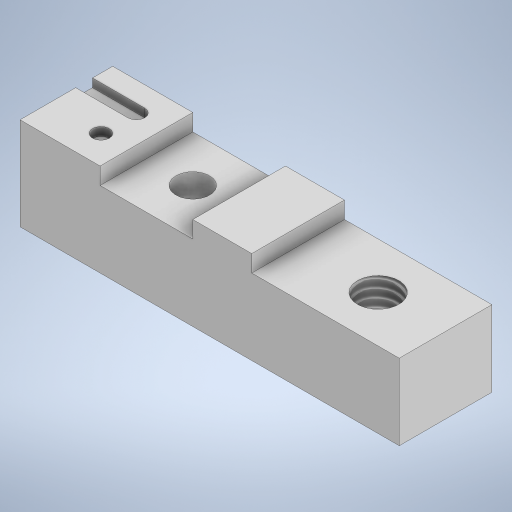
# Autodesk Inventor part: Hudson 1-55
Saved by Autodesk Inventor 2024.2 (Build 282272000, 272)
## iProperties
Created: 2024-10-06
Part Number: Hudson 1-55
Material: Genérico
Document SubType Name: Modeling
Designer: Monica Mora
Density: 1 g/cm^3
Appearance: Valor por defecto
Author: Monica Mora
Autodesk Inventor part; units mm, degrees
ref_plane "YZ Plane" through (0, 0, 0) normal (1, 0, 0) x (0, 1, 0)
ref_plane "XZ Plane" through (0, 0, 0) normal (0, 1, 0) x (-1, 0, 0)
ref_plane "XY Plane" through (0, 0, 0) normal (0, 0, 1) x (1, 0, 0)
sketch "Boceto1" plane through (0, 0, 0) normal (0, 0, 1) x (1, 0, 0)
  line L0 (0, 0) -> (-45, 0)
  line L1 (-45, 0) -> (-45, 11)
  line L2 (0, 9) -> (0, 0)
  line L3 (-35.5, 11) -> (-35.5, 9)
  line L4 (-35.5, 9) -> (-24.5, 9)
  line L5 (-24.5, 9) -> (-24.5, 11)
  line L6 (-17.5, 11) -> (-17.5, 9)
  line L7 (-17.5, 9) -> (0, 9)
  line L8 (-45, 11) -> (-35.5, 11)
  line L9 (-24.5, 11) -> (-17.5, 11)
  dimension "d0" = 9
  dimension "d1" = 11
  dimension "d2" = 9.5
  dimension "d3" = 7
  dimension "d4" = 17.5
  dimension "d5" = 11
  dimension "d6" = 2
  dimension "d7" = 2
  constraints: 20 end point, 5 perpendicular, 4 parallel, 2 point on line, 1 horizontal
  measures "d0" distance between parallel lines of L0 L7
  measures "d1" distance of L0.end L1.end
  measures "d2" distance of L1.end L3.start
  measures "d3" distance of L5.end L6.start
  measures "d4" distance of L6.end L2.start
  measures "d5" distance of L3.end L4.end
  measures "d6" distance of L3.start L3.end
  measures "d7" distance of L4.end L5.end
extrude "Extrusión1" add sketch "Boceto1" along normal blind 11
sketch "Boceto2" plane through (-45, 0, 0) normal (0, -1, 0) x (1, 0, 0)
  line L0 (0, 0) -> (45, 0) projected
  line L1 (45, 0) -> (45, 11) projected
  line L2 (0, 11) -> (45, 11) projected
  line L3 (0, 0) -> (0, 11) projected
  line L4 (45, 5.5) -> (0, 5.5) construction
  line L5 (45, 11) -> (27.5, 11) projected
  line L6 (37, 11) -> (37, 0) construction
  line L7 (15, 11) -> (15, 0) construction
  line L8 (0, 0) -> (45, 0) projected
  circle A0 centre (37, 5.5) radius 2.85
  circle A1 centre (15, 5.5) radius 4.5
  circle A2 centre (15, 5.5) radius 2
  dimension "d10" = 8
  dimension "d11" = 22
  dimension "d12" = 9
  dimension "d13" = 4
  dimension "d14" = 5.7
  constraints: 6 end point, 4 midpoint, 4 point on line, 3 centre point, 2 perpendicular, 1 coincident
  measures "d10" distance between parallel lines of L6 L1
  measures "d11" distance between parallel lines of L7 L6
  measures "d12" diameter of A1
  measures "d13" diameter of A2
  measures "d14" diameter of A0
hole "Agujero1" at (-8, 0, 5.5) direction (0, 1, 0) diameter 4.917 end through all thread size "M6x1" class "6H" standard "ANSI Metric M Profile"
hole "Agujero2" at (-30, 0, 5.5) direction (0, 1, 0) diameter 4 end through all counterbore diameter 9 counterbore depth 4.6
sketch "Boceto3" plane through (-45, 11, 0) normal (0, 1, 0) x (1, 0, 0)
  line L0 (9.5, 0) -> (0, 0) projected
  line L1 (0, 0) -> (0, -11) projected
  line L2 (9.5, -11) -> (0, -11) projected
  line L3 (9.5, 0) -> (9.5, -11) projected
  line L4 (6.2, -3.4) -> (-0.5191, -3.4) construction
  line L5 (6.2, -4.4) -> (-0.5191, -4.4)
  line L6 (-0.5191, -2.4) -> (6.2, -2.4)
  arc A0 (6.2, -4.4) -> (6.2, -2.4) centre (6.2, -3.4) ccw
  arc A1 (-0.5191, -2.4) -> (-0.5191, -4.4) centre (-0.5191, -3.4) ccw
  line L7 (9.5, -5.5) -> (0, -5.5) construction
  circle A2 centre (6.2, -7.6) radius 1
  point P0 (45, 0)
  point P1 (2.8405, -3.4)
  dimension "d29" = 2.1
  dimension "d30" = 2
  dimension "d31" = 6.2
  dimension "d32" = 2.1
  dimension "d33" = 2
  dimension "d34" = 6.2
  constraints: 10 end point, 4 point on circle, 4 tangent, 3 centre point, 3 midpoint, 1 parallel, 1 perpendicular
  measures "d29" distance between parallel lines of L7 L4
  measures "d30" distance between parallel lines of L6 L5
  measures "d31" distance from line of L1 L4.start
  measures "d32" distance from line of L7 A2.centre
  measures "d33" diameter of A2
  measures "d34" distance from line of L1 A2.centre
extrude "Extrusión2" cut sketch "Boceto3" against normal blind 1 contours L6 A0 L5 L1 | L1 L5 A1 L6 | A2
sketch "Boceto4" plane through (-45, 0, 0) normal (-1, 0, 0) x (0, 0, 1)
  line L0 (4.4, 11) -> (4.4, 10) projected
  line L1 (4.4, 10) -> (2.4, 10) projected
  line L2 (2.4, 10) -> (2.4, 11) projected
  line L3 (0, 11) -> (2.4, 11) projected
  line L4 (0, 11) -> (0, 0) projected
  line L5 (0, 0) -> (11, 0) projected
  line L6 (11, 11) -> (11, 0) projected
  line L7 (4.4, 11) -> (11, 11) projected
  line L8 (11, 5.5) -> (0, 5.5) construction
  line L9 (0, 11) -> (0, 0) projected
  line L10 (5.5, 0) -> (5.5, 11) construction
  point P0 (5.5, 5.5)
  constraints: 4 end point, 4 midpoint, 1 perpendicular, 1 point on line
hole "Agujero3" at (-45, 5.5, 5.5) direction (1, 0, 0) diameter 6.647 depth 8 thread size "M8x1.25" class "6H" standard "ANSI Metric M Profile"
